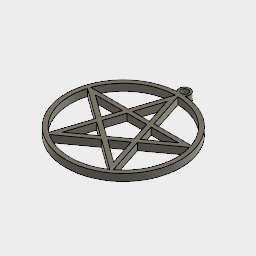
999_1 v0 (Autodesk Fusion 360 design; units mm, degrees)
Autodesk Fusion 360 part; units mm, degrees
sketch "草图1" plane through (0, 0, 0) normal (0, 1, 0) x (1, 0, 0)
  line L0 (-14.7524, -4.7933) -> (-36.0595, 10.6872)
  circle A0 centre (0, 0) radius 40.6099
  line L1 (-5.9631, 12.5492) -> (0, 30.9017)
  line L2 (-9.1175, 12.5492) -> (-0.9789, 37.5972)
  line L3 (-35.4545, 12.5492) -> (-9.1175, 12.5492)
  line L4 (-29.3893, 9.5492) -> (-10.0923, 9.5492)
  line L5 (-13.7777, -1.7933) -> (-29.3893, 9.5492)
  line L6 (-18.1636, -25) -> (-12.2005, -6.6475)
  line L7 (-11.2257, -3.6475) -> (-6.9379, 9.5492)
  line L8 (-22.891, -29.8414) -> (-14.7524, -4.7933)
  line L9 (-13.7777, -1.7933) -> (-10.0923, 9.5492)
  line L10 (29.3893, 9.5492) -> (13.7777, -1.7933)
  line L11 (36.0595, 10.6872) -> (14.7524, -4.7933)
  line L12 (12.2005, -6.6475) -> (2.552, -13.6575)
  line L13 (0, -15.5116) -> (-21.3071, -30.9921)
  line L14 (18.1636, -25) -> (2.552, -13.6575)
  line L15 (0, -11.8034) -> (-11.2257, -3.6475)
  line L16 (21.3071, -30.9921) -> (0, -15.5116)
  line L17 (-2.552, -13.6575) -> (-12.2005, -6.6475)
  line L18 (11.2257, -3.6475) -> (0, -11.8034)
  line L19 (-2.552, -13.6575) -> (-18.1636, -25)
  line L20 (14.7524, -4.7933) -> (22.891, -29.8414)
  line L21 (0.9789, 37.5972) -> (9.1175, 12.5492)
  line L22 (10.0923, 9.5492) -> (13.7777, -1.7933)
  line L23 (0, 30.9017) -> (5.9631, 12.5492)
  line L24 (-6.9379, 9.5492) -> (6.9379, 9.5492)
  line L25 (10.0923, 9.5492) -> (29.3893, 9.5492)
  line L26 (-5.9631, 12.5492) -> (5.9631, 12.5492)
  line L27 (9.1175, 12.5492) -> (35.4545, 12.5492)
  line L28 (6.9379, 9.5492) -> (11.2257, -3.6475)
  line L29 (12.2005, -6.6475) -> (18.1636, -25)
  arc A1 (-0.9789, 37.5972) -> (-35.4545, 12.5492) centre (0, 0) ccw
  arc A2 (35.4545, 12.5492) -> (0.9789, 37.5972) centre (0, 0) ccw
  arc A3 (22.891, -29.8414) -> (36.0595, 10.6872) centre (0, 0) ccw
  arc A4 (-36.0595, 10.6872) -> (-22.891, -29.8414) centre (0, 0) ccw
  arc A5 (-21.3071, -30.9921) -> (21.3071, -30.9921) centre (0, 0) ccw
extrude "拉伸1" add sketch "草图1" along normal blind 5 makes body 1
sketch "草图2" plane through (0, 5, 0) normal (0, 1, 0) x (-1, 0, 0)
  arc A0 (21.3071, 30.9921) -> (-21.3071, 30.9921) centre (0, 0) ccw
  line L0 (21.3071, 30.9921) -> (0, 15.5116)
  line L1 (0, 15.5116) -> (-21.3071, 30.9921)
  arc A1 (-22.891, 29.8414) -> (-36.0595, -10.6872) centre (0, 0) ccw
  line L2 (-22.891, 29.8414) -> (-14.7524, 4.7933)
  line L3 (-14.7524, 4.7933) -> (-36.0595, -10.6872)
  arc A2 (-35.4545, -12.5492) -> (-0.9789, -37.5972) centre (0, 0) ccw
  line L4 (-35.4545, -12.5492) -> (-9.1175, -12.5492)
  line L5 (-9.1175, -12.5492) -> (-0.9789, -37.5972)
  arc A3 (36.0595, -10.6872) -> (22.891, 29.8414) centre (0, 0) ccw
  line L6 (36.0595, -10.6872) -> (14.7524, 4.7933)
  line L7 (14.7524, 4.7933) -> (22.891, 29.8414)
  line L8 (6.9379, -9.5492) -> (-6.9379, -9.5492)
  line L9 (-6.9379, -9.5492) -> (-11.2257, 3.6475)
  line L10 (-11.2257, 3.6475) -> (0, 11.8034)
  line L11 (0, 11.8034) -> (11.2257, 3.6475)
  line L12 (11.2257, 3.6475) -> (6.9379, -9.5492)
  line L13 (-2.552, 13.6575) -> (-12.2005, 6.6475)
  line L14 (-12.2005, 6.6475) -> (-18.1636, 25)
  line L15 (-18.1636, 25) -> (-2.552, 13.6575)
  arc A4 (0.9789, -37.5972) -> (35.4545, -12.5492) centre (0, 0) ccw
  line L16 (0.9789, -37.5972) -> (9.1175, -12.5492)
  line L17 (9.1175, -12.5492) -> (35.4545, -12.5492)
  line L18 (5.9631, -12.5492) -> (0, -30.9017)
  line L19 (0, -30.9017) -> (-5.9631, -12.5492)
  line L20 (-5.9631, -12.5492) -> (5.9631, -12.5492)
  line L21 (-13.7777, 1.7933) -> (-10.0923, -9.5492)
  line L22 (-10.0923, -9.5492) -> (-29.3893, -9.5492)
  line L23 (-29.3893, -9.5492) -> (-13.7777, 1.7933)
  line L24 (12.2005, 6.6475) -> (2.552, 13.6575)
  line L25 (2.552, 13.6575) -> (18.1636, 25)
  line L26 (18.1636, 25) -> (12.2005, 6.6475)
  line L27 (13.7777, 1.7933) -> (29.3893, -9.5492)
  line L28 (29.3893, -9.5492) -> (10.0923, -9.5492)
  line L29 (10.0923, -9.5492) -> (13.7777, 1.7933)
  circle A5 centre (0, 0) radius 40.6099
  circle A6 centre (55, 0) radius 2.5
  circle A7 centre (55, 0) radius 4
  dimension "d5" = 8
  measures "d5" diameter of A7
extrude "拉伸2" add sketch "草图2" along normal blind 5 separate body contours A7 makes body 2
move_body "移动1" bodies 2 to x (1, 0, 0) y (0, 1, 0) z (0, 0, 1) at (0, -5, 0)
move_body "移动2" bodies 2 to x (1, 0, 0) y (0, 1, 0) z (0, 0, 1) at (55.2046, 0, -43.1842)
combine "合并1" operation add target body 1 tool bodies 2
